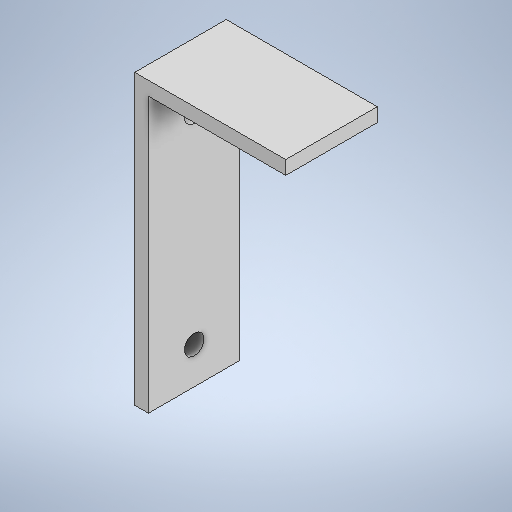
# Autodesk Inventor part: BedBeltMount1
Saved by Autodesk Inventor 2025.2 (Build 292293000, 293)
## iProperties
Created: 2025-07-28
Part Number: BedBeltMount1
Material: Generic
Document SubType Name: Modeling
Designer: Simon
Density: 1 g/cm^3
Appearance: Default
Author: Simon
Autodesk Inventor part; units mm, degrees
ref_plane "YZ Plane" through (0, 0, 0) normal (1, 0, 0) x (0, 1, 0)
ref_plane "XZ Plane" through (0, 0, 0) normal (0, 1, 0) x (-1, 0, 0)
ref_plane "XY Plane" through (0, 0, 0) normal (0, 0, 1) x (1, 0, 0)
sketch "Sketch1" plane through (0, 0, 0) normal (0, 0, 1) x (1, 0, 0)
  line L0 (0, 0) -> (-30, 0)
  line L1 (-30, 0) -> (-30, -60)
  line L2 (0, 0) -> (-30, 0)
  line L3 (-30, 0) -> (-30, 3)
  line L4 (-30, 3) -> (0, 3)
  line L5 (0, 3) -> (0, 0)
  line L6 (-30, -60) -> (-33, -60)
  line L7 (-33, -60) -> (-33, 0)
  line L8 (-33, 0) -> (-30, 0)
  line L9 (-30, 0) -> (-30, -60)
  line L10 (-30, 3) -> (-33, 3)
  line L11 (-33, 3) -> (-33, 0)
  line L12 (-33, 0) -> (-30, 0)
  line L13 (-30, 0) -> (-30, 3)
  dimension "d0" = 30
  dimension "d1" = 60
  dimension "d2" = 3
  dimension "d3" = 3
  constraints: 28 end point, 6 parallel, 4 horizontal, 4 perpendicular, 1 point on line
  measures "d0" distance of L0.start L0.end
  measures "d1" distance of L0.end L1.end
  measures "d2" distance of L2.end L3.end
  measures "d3" distance of L7.end L8.end
extrude "Extrusion1" add sketch "Sketch1" along normal blind 20
sketch "Sketch2" plane through (-30, -60, 0) normal (1, 0, 0) x (0, 0, -1)
  line L0 (0, 63) -> (0, 0) projected
  line L1 (-20, 63) -> (-20, 0) projected
  line L2 (0, 0) -> (-20, 0)
  line L3 (-20, 0) -> (-20, 60)
  line L4 (-20, 60) -> (0, 60)
  line L5 (0, 60) -> (0, 0)
  line L6 (-10, 0) -> (-10, 8)
  line L7 (-10, 60) -> (-10, 52)
  circle A0 centre (-10, 52) radius 2.15
  circle A1 centre (-10, 8) radius 2.15
  dimension "d6" = 8
  dimension "d7" = 8
  dimension "d8" = 4.3
  dimension "d9" = 4.3
  constraints: 12 end point, 2 centre point, 2 coincident, 2 midpoint, 2 parallel, 2 vertical, 1 horizontal, 1 perpendicular, 1 point on line
  measures "d6" distance of L6.start L6.end
  measures "d7" distance of L7.start L7.end
  measures "d8" diameter of A0
  measures "d9" diameter of A1
extrude "Extrusion2" cut sketch "Sketch2" against normal through all contours A0 | A1
body "Solid1"
